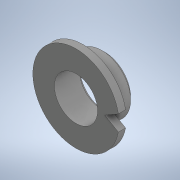
# Autodesk Inventor part: tuleja_TUF106040
Saved by Autodesk Inventor 2020.3 (Build 243373000, 373)
## iProperties
Created: 2021-10-24
Part Number: tuleja_TUF106040
Material: Ogólny
Document SubType Name: Modeling
Designer: patry
Density: 1 g/cm^3
Appearance: Czarny
Author: patry
Autodesk Inventor part; units mm, degrees
ref_plane "YZ Plane" through (0, 0, 0) normal (1, 0, 0) x (0, 1, 0)
ref_plane "XZ Plane" through (0, 0, 0) normal (0, 1, 0) x (-1, 0, 0)
ref_plane "XY Plane" through (0, 0, 0) normal (0, 0, 1) x (1, 0, 0)
sketch "Szkic1" plane through (0, 0, 0) normal (0, 0, 1) x (1, 0, 0)
  circle A0 centre (0, 0) radius 3
  circle A1 centre (0, 0) radius 4
  circle A2 centre (0, 0) radius 6
  dimension "d0" = 6
  dimension "d1" = 8
  dimension "d2" = 12
  constraints: 3 centre point, 3 coincident
  measures "d0" diameter of A0
  measures "d1" diameter of A1
  measures "d2" diameter of A2
extrude "Wyciągnięcie proste1" add sketch "Szkic1" along normal blind 1 contours A1 | A2
extrude "Wyciągnięcie proste2" add sketch "Szkic1" against normal blind 3 contours A1
sketch "Szkic2" plane through (0, 0, 1) normal (0, 0, 1) x (1, 0, 0)
  circle A0 centre (0, 0) radius 4 projected
  line L0 (4, 0) -> (5.899, 1.0964)
  circle A1 centre (0, 0) radius 6 projected
  line L1 (4, 0) -> (5.9306, -1.1146)
  line L2 (4, 0) -> (6, 0) construction
  circle A2 centre (0, 0) radius 6 construction
  circle A3 centre (0, 0) radius 6 construction
  circle A4 centre (0, 0) radius 3 construction
  point P0 (5.899, -1.0964)
  dimension "d7" = 60
  dimension "d8" = 30
  constraints: 6 end point, 2 point on circle, 1 horizontal, 1 horizontal alignment, 1 other
  measures "d7" angle of L1 L0
  measures "d8" angle of L0 L2
extrude "Wyciągnięcie proste3" cut sketch "Szkic2" against normal blind 10 contours L0 A1 L1 picked at (5.2847, 0.6099)
chamfer "Faza1" distance 0.4 angle 45 1 edges at (-4, 0, -3)
chamfer "Faza2" distance 0.5 angle 45 1 edges at (-3, 0, -3)
equation "\"d8\" = 0.5 * d7"
